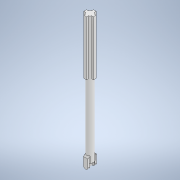
# Autodesk Inventor part: Lower Arm
Saved by Autodesk Inventor 2022 (Build 260153000, 153)
## iProperties
Created: 2022-03-03
Part Number: Lower Arm
Material: Generic
Document SubType Name: Modeling
Designer: Dahway
Density: 1 g/cm^3
Appearance: PLA
Author: Dahway
Autodesk Inventor part; units mm, degrees
ref_plane "YZ Plane" through (0, 0, 0) normal (1, 0, 0) x (0, 1, 0)
ref_plane "XZ Plane" through (0, 0, 0) normal (0, 1, 0) x (-1, 0, 0)
ref_plane "XY Plane" through (0, 0, 0) normal (0, 0, 1) x (1, 0, 0)
sketch "Sketch7" plane through (0, 0, 0) normal (0, 1, 0) x (-1, 0, 0)
  circle A0 centre (0, 0) radius 3.75
  dimension "d71" = 7.5
  constraints: 1 centre point, 1 coincident
  measures "d71" diameter of A0
extrude "Extrusion7" add sketch "Sketch7" along normal blind 130
sketch "Sketch8" plane through (0, 130, 0) normal (0, 1, 0) x (1, 0, 0)
  line L0 (-5.25, -1.5) -> (-2.25, -1.5)
  line L1 (-2.25, -1.5) -> (-2.25, 1.5)
  line L2 (-2.25, 1.5) -> (-5.25, 1.5)
  line L3 (-5.25, 1.5) -> (-5.25, -1.5)
  circle A0 centre (0, 0) radius 3.75 projected
  line L4 (-5.25, -1.5) -> (-2.25, 1.5) construction
  line L5 (-2.25, -1.5) -> (-5.25, 1.5) construction
  line L6 (1.5, 2.25) -> (-1.5, 2.25)
  line L7 (-1.5, 2.25) -> (-1.5, 5.25)
  line L8 (-1.5, 5.25) -> (1.5, 5.25)
  line L9 (1.5, 5.25) -> (1.5, 2.25)
  line L10 (1.5, 2.25) -> (-1.5, 5.25) construction
  line L11 (-1.5, 2.25) -> (1.5, 5.25) construction
  line L12 (2.25, -1.5) -> (5.25, -1.5)
  line L13 (5.25, -1.5) -> (5.25, 1.5)
  line L14 (5.25, 1.5) -> (2.25, 1.5)
  line L15 (2.25, 1.5) -> (2.25, -1.5)
  line L16 (2.25, -1.5) -> (5.25, 1.5) construction
  line L17 (5.25, -1.5) -> (2.25, 1.5) construction
  line L18 (-1.5, -5.25) -> (1.5, -5.25)
  line L19 (1.5, -5.25) -> (1.5, -2.25)
  line L20 (1.5, -2.25) -> (-1.5, -2.25)
  line L21 (-1.5, -2.25) -> (-1.5, -5.25)
  line L22 (-1.5, -5.25) -> (1.5, -2.25) construction
  line L23 (1.5, -5.25) -> (-1.5, -2.25) construction
  point P0 (-3.75, 0)
  point P1 (0, 3.75)
  point P2 (3.75, 0)
  point P3 (0, -3.75)
  point P4 (3.4369, 1.5)
  point P5 (3.4369, -1.5)
  point P6 (-1.5, 3.4369)
  point P7 (1.5, 3.4369)
  point P8 (-3.4369, -1.5)
  point P9 (-3.4369, 1.5)
  point P10 (1.5, -3.4369)
  point P11 (-1.5, -3.4369)
  dimension "d74" = 3
  dimension "d75" = 3
  dimension "d76" = 3
  dimension "d77" = 3
  dimension "d78" = 3
  dimension "d79" = 3
  dimension "d80" = 3
  dimension "d81" = 3
  constraints: 48 end point, 8 midpoint, 8 parallel, 4 horizontal, 4 perpendicular, 4 point on circle, 3 point on line
  measures "d74" distance of L2.end L1.end
  measures "d75" distance of L1.end L0.end
  measures "d76" distance of L7.end L8.end
  measures "d77" distance of L6.end L7.end
  measures "d78" distance of L14.end L13.end
  measures "d79" distance of L13.end L12.end
  measures "d80" distance of L20.end L19.end
  measures "d81" distance of L19.end L18.end
extrude "Extrusion8" add sketch "Sketch8" along normal blind 10 and the other way blind 50
sketch "Sketch9" plane through (0, 0, 0) normal (0, -1, 0) x (1, 0, 0)
  line L0 (-2.5, 4.75) -> (2.5, 4.75)
  line L1 (2.5, 4.75) -> (2.5, 2.75)
  line L2 (2.5, 2.75) -> (-2.5, 2.75)
  line L3 (-2.5, 2.75) -> (-2.5, 4.75)
  line L4 (-2.5, 4.75) -> (2.5, 2.75) construction
  line L5 (2.5, 4.75) -> (-2.5, 2.75) construction
  line L6 (-5.25, 1.5) -> (-5.25, -1.5) projected
  line L7 (-2.5, -2.75) -> (2.5, -2.75)
  line L8 (2.5, -2.75) -> (2.5, -4.75)
  line L9 (2.5, -4.75) -> (-2.5, -4.75)
  line L10 (-2.5, -4.75) -> (-2.5, -2.75)
  line L11 (-2.5, -2.75) -> (2.5, -4.75) construction
  line L12 (2.5, -2.75) -> (-2.5, -4.75) construction
  point P0 (0, 0)
  point P1 (0, 3.75)
  point P2 (0, -3.75)
  dimension "d86" = 5
  dimension "d87" = 2
  dimension "d88" = 2.75
  dimension "d89" = 2.75
  dimension "d90" = 2
  dimension "d91" = 5.5
  dimension "d92" = 2.75
  constraints: 24 end point, 4 midpoint, 4 parallel, 2 horizontal, 2 perpendicular
  measures "d86" distance of L1.end L2.end
  measures "d87" distance of L0.end L1.end
  measures "d88" distance from line of point (0, 0) L2
  measures "d89" distance between parallel lines of L6 L3
  measures "d90" distance of L7.end L8.end
  measures "d91" distance between parallel lines of L7 L2
  measures "d92" distance between parallel lines of L6 L10
extrude "Extrusion9" add sketch "Sketch9" along normal blind 6 and the other way blind 5
fillet "Fillet1" radius 2 2 edges at (0, 5, 3.75) (0, 5, -3.75)
fillet "Fillet3" radius 1 8 edges at (2.5, 2.5, -2.7951) (2.5, 5.9727, -2.7951) (-2.5, 5.9727, -2.7951) (-2.5, 2.5, -2.7951) (-2.5, 2.5, 2.7951) (-2.5, 5.9727, 2.7951) (2.5, 5.9727, 2.7951) (2.5, 2.5, 2.7951)
fillet "Fillet5" radius 1 2 edges at (0, 0, -2.75) (0, 0, 2.75)
fillet "Fillet6" radius 0.5 12 edges at (-2.5, 0, 2.25) (-2.5, 0, 2.7725) (-2.5, 0, 3.0032) (-2.5, 0, -2.7725) (-2.5, 0, -2.25) (-2.5, 0, -3.0032) (2.5, 0, -2.7725) (2.5, 0, -2.25) (2.5, 0, -3.0032) (2.5, 0, 2.7725) (2.5, 0, 2.25) (2.5, 0, 3.0032)
fillet "Fillet7" radius 2.5 4 edges at (2.5, -6, -3.75) (-2.5, -6, -3.75) (2.5, -6, 3.75) (-2.5, -6, 3.75)
sketch "Sketch11" plane through (-2.5, -1, -2.75) normal (0, 0, 1) x (1, 0, 0)
  circle A0 centre (2.5, -2.5) radius 1.5
  line L0 (3, -5) -> (2, -5) projected
  line L1 (5, 0) -> (5, -2.5) projected
  point P0 (2.5, 1)
  dimension "d109" = 3
  dimension "d110" = 2.5
  dimension "d111" = 2.5
  constraints: 1 centre point
  measures "d109" diameter of A0
  measures "d110" distance from line of L0 A0.centre
  measures "d111" distance from line of L1 A0.centre
extrude "Extrusion11" add sketch "Sketch11" along normal up to surface (5.5 mm away)
fillet "Fillet8" radius 1 2 edges at (-1.5, -3.5, 2.75) (-1.5, -3.5, -2.75)
body "Solid4"
